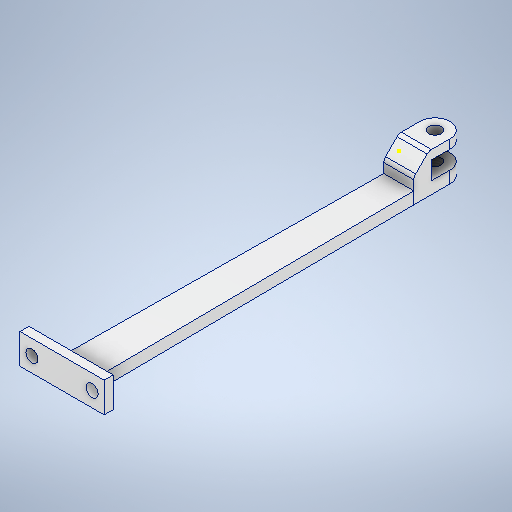
# Autodesk Inventor part: 205
Saved by Autodesk Inventor 2025.1 (Build 291241000, 241)
## iProperties
Created: 2024-06-12
Part Number: 205
Material: Aluminium 6061
Document SubType Name: Modeling
Designer: ffogue
Density: 2.7 g/cm^3
Appearance: Aluminium - flach
Author: ffogue
Autodesk Inventor part; units mm, degrees
ref_plane "YZ Plane" through (0, 0, 0) normal (1, 0, 0) x (0, 1, 0)
ref_plane "XZ Plane" through (0, 0, 0) normal (0, 1, 0) x (-1, 0, 0)
ref_plane "XY Plane" through (0, 0, 0) normal (0, 0, 1) x (1, 0, 0)
sketch "Skizze1" plane through (0, 0, 0) normal (0, 1, 0) x (-1, 0, 0)
  point P0 (0, 0)
sketch "Skizze2" plane through (0, 0, 0) normal (1, 0, 0) x (0, 1, 0)
  line L0 (5, 0) -> (17, 0)
  line L1 (17, -13) -> (0, -13)
  line L2 (0, -13) -> (0, -5)
  line L3 (5, 0) -> (0, -5)
  line L4 (17, -3) -> (6, -3)
  line L5 (6, -3) -> (6, -9)
  line L6 (6, -9) -> (17, -9)
  line L7 (17, 0) -> (17, -3)
  line L8 (17, -9) -> (17, -13)
  point P0 (0, 0)
  point P1 (17, -11)
  dimension "d1" = 13
  dimension "d2" = 5
  dimension "d5" = 3
  dimension "d6" = 4
  dimension "d7" = 11
  dimension "d8" = 12
  dimension "d9" = 17
  constraints: 18 end point, 4 perpendicular, 3 parallel, 2 horizontal, 1 horizontal alignment, 1 midpoint, 1 vertical
  measures "d1" distance between parallel lines of L0 L1
  measures "d2" horizontal distance of L0.start L2.end
  measures "d5" distance between parallel lines of L4 L0
  measures "d6" distance between parallel lines of L1 L6
  measures "d7" distance from line of L4.start L5
  measures "d8" horizontal distance of point (17, -11) L0.start
  measures "d9" distance between parallel lines of L2 L8
extrude "Extrusion1" add sketch "Skizze2" along normal mid plane 10
fillet "Rundung1" radius 5 2 edges at (5, 17, -1.5) (-5, 17, -1.5)
fillet "Rundung2" radius 5 2 edges at (5, 17, -11) (-5, 17, -11)
sketch "Skizze4" plane through (5, 0, -13) normal (0, 0, -1) x (-1, 0, 0)
  arc A0 (10, 12) -> (0, 12) centre (5, 12) ccw projected
  point P0 (5, 0)
  constraints: 1 coincident
hole "Bohrung1" at (0, 12, -13) direction (0, 0, 1) diameter 4.134 depth 4 thread size "M5x0.8" class "6H" standard "ISO Metric profile"
sketch "Skizze5" plane through (-5, 5, 0) normal (0, 0, 1) x (1, 0, 0)
  arc A0 (10, 7) -> (0, 7) centre (5, 7) ccw projected
  point P0 (5, -5)
  constraints: 1 coincident
hole "Bohrung2" at (0, 12, 0) direction (0, 0, -1) diameter 4.134 depth 3 thread size "M5x0.8" class "6H" standard "ISO Metric profile"
sketch "Skizze6" plane through (5, 0, -13) normal (0, 0, -1) x (-1, 0, 0)
  line L0 (0, 0) -> (-1, -109)
  line L1 (10, 0) -> (0, 0) projected
  line L2 (10, 0) -> (11, -109)
  line L3 (5, 0) -> (5, -23.6685) construction
  line L4 (-1, -109) -> (11, -109)
  circle A0 centre (5, 12) radius 2.067 projected
  dimension "d29" = 12
  dimension "d30" = 121
  constraints: 8 end point, 1 horizontal, 1 symmetric about line, 1 vertical
  measures "d29" distance of L2.end L0.end
  measures "d30" distance from line of L4 A0.centre
extrude "Extrusion2" add sketch "Skizze6" against normal blind 4 contours L1 L2 L4 L0
fillet "Rundung3" radius 2 2 edges at (0, 0, -5) (0, 5, 0)
sketch "Skizze7" plane through (0, 12, -13) normal (0, 0, -1) x (-1, 0, 0)
  line L0 (-14, -121) -> (14, -121)
  line L1 (14, -121) -> (14, -124)
  line L2 (14, -124) -> (-14, -124)
  line L3 (-14, -124) -> (-14, -121)
  line L4 (-6, -121) -> (6, -121) projected
  point P0 (0, -12)
  point P1 (0, -124)
  point P2 (0, -121)
  point P3 (0, -121)
  dimension "d34" = 28
  dimension "d35" = 3
  constraints: 8 end point, 4 midpoint, 2 parallel, 1 horizontal, 1 perpendicular, 1 vertical alignment
  measures "d34" distance of L1.end L2.end
  measures "d35" distance between parallel lines of L2 L0
extrude "Extrusion3" add sketch "Skizze7" against normal blind 10
fillet "Rundung4" radius 0.5 3 edges at (6, -109, -11) (-6, -109, -11) (0, -109, -9)
sketch "Skizze8" plane through (-14, -109, -3) normal (0, 1, 0) x (1, 0, 0)
  line L0 (9, 10) -> (19, 10) projected
  line L1 (0, 10) -> (0, 0) projected
  point P0 (14, -3)
  point P1 (4, 5)
  point P2 (24, 5)
  point P3 (14, 10)
  point P4 (14, 10)
  point P5 (0, 5)
  dimension "d46" = 10
  dimension "d47" = 10
  constraints: 3 midpoint, 2 horizontal alignment
  measures "d46" horizontal distance of point (14, 10) point (4, 5)
  measures "d47" horizontal distance of point (24, 5) point (14, 10)
hole "Bohrung3" at (-10, -109, -8) at (10, -109, -8) direction (0, -1, 0) diameter 4 depth 3
